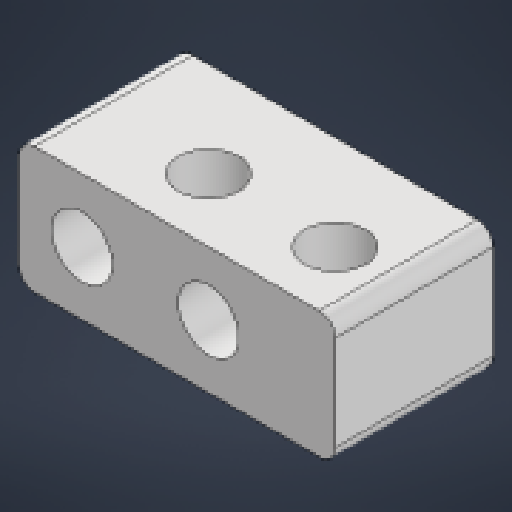
# Autodesk Inventor part: 3DPRINT,LEFT,NUT-BLOCK
Saved by Autodesk Inventor 2026.1 (Build 301233020, 233B)
## iProperties
Created: 2026-04-01
Part Number: 3DPRINT,LEFT,NUT-BLOCK
Material: Nylon 6/6
Document SubType Name: Modeling
Designer: Owen L
Density: 1.13 g/cm^3
Appearance: Smooth - Black
Author: Owen L
Autodesk Inventor part; units mm, degrees
ref_plane "YZ Plane" through (0, 0, 0) normal (1, 0, 0) x (0, 1, 0)
ref_plane "XZ Plane" through (0, 0, 0) normal (0, 1, 0) x (-1, 0, 0)
ref_plane "XY Plane" through (0, 0, 0) normal (0, 0, 1) x (1, 0, 0)
sketch "Sketch1" plane through (0, 0, 0) normal (0, 0, 1) x (1, 0, 0)
  line L0 (15.875, -6.35) -> (-15.875, -6.35)
  line L1 (-15.875, -6.35) -> (-15.875, 6.35)
  line L2 (-15.875, 6.35) -> (15.875, 6.35)
  line L3 (15.875, 6.35) -> (15.875, -6.35)
  line L4 (15.875, -6.35) -> (-15.875, 6.35) construction
  line L5 (-15.875, -6.35) -> (15.875, 6.35) construction
  point P0 (0, 0)
  dimension "d0" = 31.75
  dimension "d1" = 12.7
  constraints: 12 end point, 2 midpoint, 2 parallel, 1 horizontal, 1 perpendicular
  measures "d0" distance of L1.end L2.end
  measures "d1" distance of L0.end L1.end
extrude "Extrusion1" add sketch "Sketch1" along normal blind 15.875
sketch "Sketch2" plane through (0, 0, 0) normal (0, 0, -1) x (-1, 0, 0)
  line L0 (15.875, 6.35) -> (15.875, -6.35) projected
  point P0 (0, 0)
  point P1 (9.525, 0)
  point P2 (-3.175, 0)
  dimension "d4" = 12.7
  dimension "d5" = 6.35
  constraints: 2 horizontal alignment
  measures "d4" distance of point (-3.175, 0) point (9.525, 0)
  measures "d5" distance from line of L0 point (9.525, 0)
hole "Hole1" at (-9.525, 0, 0) at (3.175, 0, 0) direction (0, 0, 1) diameter 6.096 end through all
sketch "Sketch3" plane through (-15.875, -6.35, 0) normal (0, -1, 0) x (1, 0, 0)
  line L0 (0, 0) -> (0, 15.875) projected
  line L1 (0, 0) -> (31.75, 0) projected
  point P0 (15.875, 0)
  point P1 (12.7, 9.525)
  point P2 (25.4, 9.525)
  dimension "d13" = 12.7
  dimension "d14" = 12.7
  dimension "d15" = 9.525
  constraints: 1 horizontal alignment
  measures "d13" distance from line of L0 point (12.7, 9.525)
  measures "d14" distance of point (12.7, 9.525) point (25.4, 9.525)
  measures "d15" distance from line of L1 point (12.7, 9.525)
hole "Hole2" at (-3.175, -6.35, 9.525) at (9.525, -6.35, 9.525) direction (0, 1, 0) diameter 6.096 end through all
fillet "Fillet1" radius 1.5875 4 edges at (-15.875, -6.35, 7.9375) (-15.875, 6.35, 7.9375) (15.875, -6.35, 7.9375) (15.875, 6.35, 7.9375)
body "Solid1"
